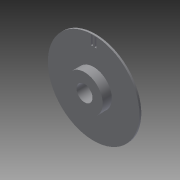
# Autodesk Inventor part: BigPositionDisk
Saved by Autodesk Inventor 2015 (Build 190159000, 159)
## iProperties
Created: 2017-01-31
Part Number: BigPositionDisk
Material: Generic
Document SubType Name: Modeling
Designer: Ernest
Density: 1 g/cm^3
Appearance: Default
Author: Ernest
Autodesk Inventor part; units mm, degrees
ref_plane "YZ Plane" through (0, 0, 0) normal (1, 0, 0) x (0, 1, 0)
ref_plane "XZ Plane" through (0, 0, 0) normal (0, 1, 0) x (-1, 0, 0)
ref_plane "XY Plane" through (0, 0, 0) normal (0, 0, 1) x (1, 0, 0)
sketch "Sketch1" plane through (0, 0, 0) normal (0, 1, 0) x (-1, 0, 0)
  circle A0 centre (0, 0) radius 25.2
  line L0 (0, 0) -> (25.2, 0)
  circle A1 centre (0, 0) radius 4.4
  dimension "d1" = 50.4
  dimension "d6" = 8.8
  constraints: 2 end point, 1 centre point, 1 horizontal, 1 horizontal alignment, 2 other
  measures "d6" diameter of A1
extrude "Extrusion1" add sketch "Sketch1" along normal blind 6
sketch "Sketch2" plane through (0, 0, 0) normal (0, -1, 0) x (1, 0, 0)
  circle A0 centre (0, 0) radius 4.4 projected
  circle A1 centre (0, 0) radius 25.2 projected
  circle A2 centre (0, 0) radius 10
  circle A3 centre (0, 0) radius 25.2
  dimension "d7" = 20
  constraints: 2 centre point, 2 coincident
  measures "d7" diameter of A2
extrude "Extrusion2" cut sketch "Sketch2" against normal blind 5 contours A1
sketch "Sketch3" plane through (0, 6, 0) normal (0, 1, 0) x (1, 0, 0)
  circle A0 centre (0, 0) radius 4.4 projected
  circle A1 centre (0, 0) radius 25.2 projected
  line L0 (0, 0) -> (0, -25.2)
  circle A2 centre (0, 0) radius 25.2 projected
  line L1 (2.2, -19.04) -> (2.2, -25.2)
  line L2 (2.2, -25.2) -> (-2.2, -25.2)
  line L3 (-2.2, -25.2) -> (-2.2, -19.04)
  line L4 (-2.2, -19.04) -> (2.2, -19.04)
  line L5 (2.2, -19.04) -> (-2.2, -25.2) construction
  line L6 (2.2, -25.2) -> (-2.2, -19.04) construction
  line L7 (1.5, -24.62) -> (0.5, -24.62)
  line L8 (0.5, -24.62) -> (0.5, -19.62)
  line L9 (0.5, -19.62) -> (1.5, -19.62)
  line L10 (1.5, -19.62) -> (1.5, -24.62)
  line L11 (-0.5, -24.62) -> (-1.5, -24.62)
  line L12 (-1.5, -24.62) -> (-1.5, -19.62)
  line L13 (-1.5, -19.62) -> (-0.5, -19.62)
  line L14 (-0.5, -19.62) -> (-0.5, -24.62)
  point P0 (0, -22.12)
  dimension "d10" = 0
  dimension "d11" = 4.4
  dimension "d12" = 6.16
  dimension "d13" = 1
  dimension "d14" = 5
  dimension "d17" = 0.58
  dimension "d22" = 2
  dimension "d23" = 0.5
  constraints: 30 end point, 7 parallel, 3 perpendicular, 3 point on line, 2 horizontal, 2 midpoint, 2 vertical alignment, 1 collinear, 1 vertical, 2 other
  measures "d10" distance from line of L0.end L2
  measures "d11" distance of L1.end L2.end
  measures "d12" distance of L2.end L3.end
  measures "d13" distance of L7.start L7.end
  measures "d14" distance of L9.end L7.start
  measures "d17" distance between parallel lines of L2 L11
  measures "d22" distance between parallel lines of L14 L10
  measures "d23" distance between parallel lines of L0 L8
extrude "Extrusion3" cut sketch "Sketch3" against normal blind 5 contours L7 L8 L9 L10 | L11 L12 L13 L14
equation "\"d17\" = -0.5 * d14 + 0.5 * d12"
equation "\"d23\" = -0.5 * d13 + 0.5 * d22"
body "Solid1"
